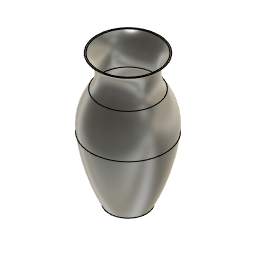
Sketch28_Final (Autodesk Fusion 360 design; units mm, degrees)
Autodesk Fusion 360 part; units mm, degrees
sketch "Sketch1" plane through (0, 0, 0) normal (0, 1, 0) x (1, 0, 0)
  line L0 (0, 0) -> (-30, 0)
  line L1 (0, -100) -> (-60, -100)
  line L2 (0, -160) -> (-45, -160)
  line L3 (0, -210) -> (-50, -210)
  arc A0 (-50, -210) -> (-45, -160) centre (-76.6667, -182.0833) ccw
  arc A1 (-60, -100) -> (-45, -160) centre (26.25, -110.3125) ccw
  arc A2 (-30, 0) -> (-60, -100) centre (242.0482, -136.1145) ccw
  line L4 (0, -210) -> (-48, -210)
  line L5 (0, -160) -> (-43, -160)
  line L6 (0, -100) -> (-58, -100)
  line L7 (0, 0) -> (-28, 0)
  arc A3 (-28.9913, -2) -> (-58, -100) centre (244.2, -136.16) ccw
  arc A4 (-58, -100) -> (-43, -160) centre (27.2134, -110.5716) ccw
  arc A5 (-48, -210) -> (-43, -160) centre (-75.8013, -181.9699) ccw
  line L8 (0, 0) -> (0, -2)
  line L9 (0, -2) -> (-28.9913, -2)
  dimension "d1" = 30
  dimension "d2" = 100
  dimension "d3" = 60
  dimension "d4" = 60
  dimension "d5" = 45
  dimension "d6" = 50
  dimension "d7" = 50
  dimension "d9" = 48
  dimension "d10" = 43
  dimension "d11" = 58
  dimension "d12" = 28
  constraint coincident L0.start L7.start
  constraint horizontal L0
  constraint tangent A0 A1
  constraint tangent A1 A2
  constraint tangent A1 A4
  constraint tangent A0 A5
  constraint perpendicular L0 L8
  constraint perpendicular L8 L9
  measures "d1" distance of L0.start L0.end
  measures "d2" distance of L0.start L1.start
  measures "d3" distance of L1.start L1.end
  measures "d4" distance of L1.start L2.start
  measures "d5" distance of L2.start L2.end
  measures "d6" distance of L2.start L3.start
  measures "d7" distance of L3.start L3.end
  measures "d9" distance of L3.start L4.end
  measures "d10" distance of L2.start L5.end
  measures "d11" distance of L1.start L6.end
  measures "d12" distance of L0.start L7.end
revolve "Revolve1" add sketch "Sketch1" angle 360 about axis through (0, 0, 1.75) along (0, 0, 1) second angle 360
